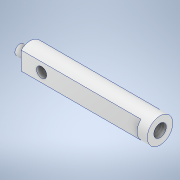
# Autodesk Inventor part: Shaft_newtest
Saved by Autodesk Inventor 2021 (Build 250183000, 183)
## iProperties
Created: 2022-02-13
Part Number: Shaft_newtest
Material: Aluminium 6061
Document SubType Name: Modeling
Designer: Timo de Vries
Density: 2.7 g/cm^3
Appearance: Aluminium - flach
Mass: 8.77035 g
Surface Area: 18.2114 cm^2
Volume: 3.24828 cm^3
Author: Timo de Vries
Autodesk Inventor part; units mm, degrees
ref_plane "YZ Plane" through (0, 0, 0) normal (1, 0, 0) x (0, 1, 0)
ref_plane "XZ Plane" through (0, 0, 0) normal (0, 1, 0) x (-1, 0, 0)
ref_plane "XY Plane" through (0, 0, 0) normal (0, 0, 1) x (1, 0, 0)
sketch "Skizze1" plane through (0, 0, 0) normal (0, 0, 1) x (1, 0, 0)
  line L0 (0, 0) -> (-67, 0)
  line L1 (-51, 5) -> (0, 5)
  line L2 (0, 5) -> (0, 0)
  line L3 (-51, 5) -> (-51, 2)
  line L4 (-51, 2) -> (-55, 2)
  line L5 (-55, 2) -> (-55, 0)
  line L6 (-56, 0) -> (-55, 0)
  dimension "d0" = 51
  dimension "d42" = 10
  dimension "d60" = 4
  dimension "d61" = 4
  constraints: 14 end point, 3 perpendicular, 2 point on line, 2 vertical, 1 horizontal, 1 parallel
  measures "d0" distance of L1.start L1.end
  measures "d42" diameter of L1 L0
  measures "d60" diameter of L4 L0
  measures "d61" distance between parallel lines of L3 L5
revolve "Umdrehung1" add sketch "Skizze1" angle 360 about axis through (0, 0, 0) along (-1, 0, 0)
sketch "Skizze3" plane through (0, 0, 0) normal (0, 1, 0) x (-1, 0, 0)
  line L0 (51, 5) -> (51, -5) construction
  line L1 (51, -5) -> (0, -5) construction
  line L2 (51, 5) -> (0, 5) construction
  line L3 (51, -5) -> (4, -5)
  line L4 (4, -5) -> (4, -3.5)
  line L5 (4, -3.5) -> (51, -3.5)
  line L6 (51, -3.5) -> (51, -5)
  line L7 (4, 5) -> (51, 5)
  line L8 (51, 5) -> (51, 3.5)
  line L9 (51, 3.5) -> (4, 3.5)
  line L10 (4, 3.5) -> (4, 5)
  line L11 (0, 5) -> (0, -5) projected
  point P0 (0, 0)
  dimension "d10" = 7
  dimension "d11" = 4
  constraints: 16 end point, 4 parallel, 3 point on line, 2 horizontal, 2 perpendicular, 1 collinear
  measures "d10" distance between parallel lines of L5 L9
  measures "d11" distance between parallel lines of L4 L11
extrude "Extrusion1" cut sketch "Skizze3" along normal through all both and the other way through all
sketch "Skizze8" plane through (-4, -3.5707, 3.5) normal (0, 0, 1) x (1, 0, 0)
  line L0 (0, 0) -> (-47, 0) construction
  line L1 (0, 7.1414) -> (0, 0) construction
  line L2 (-47, 7.1414) -> (0, 7.1414) construction
  line L3 (-47, 0) -> (-47, 7.1414) construction
  line L4 (4, -1.4293) -> (4, 8.5707) construction
  point P0 (-39, 3.5707)
  point P1 (4, 3.5707)
  dimension "d63" = 8
  constraints: 1 horizontal alignment, 1 midpoint
  measures "d63" distance from line of L3 point (-39, 3.571)
hole "Bohrung3" at (-43, 0, 3.5) direction (0, 0, -1) diameter 4 end through all
sketch "Skizze9" plane through (0, 0, 0) normal (1, 0, 0) x (0, 0, -1)
  circle A0 centre (0, 0) radius 5 construction
  constraints: 1 coincident
hole "Bohrung5" at (0, 0, 0) direction (-1, 0, 0) diameter 4.917 depth 12 tip angle 118 thread size "M6x1" class "6H" standard "ISO Metric profile"
